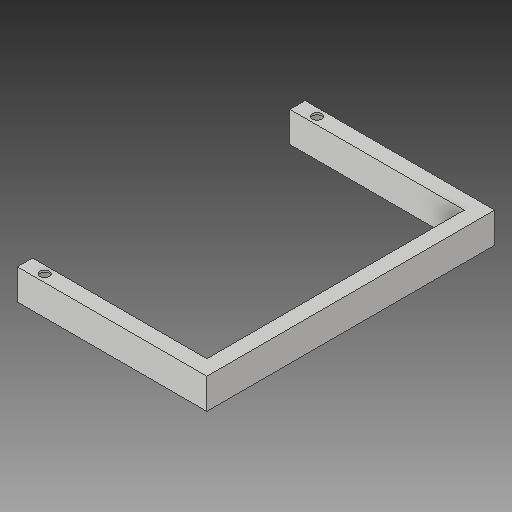
# Autodesk Inventor part: GripperFrame
Saved by Autodesk Inventor 2019 (Build 230136000, 136)
## iProperties
Created: 2018-01-17
Part Number: GripperFrame
Material: Generic
Document SubType Name: Modeling
Designer: steele
Density: 1 g/cm^3
Appearance: Default
Author: steele
Autodesk Inventor part; units mm, degrees
ref_plane "XZ Plane" through (0, 0, 0) normal (0, 1, 0) x (-1, 0, 0)
ref_plane "XY Plane" through (0, 0, 0) normal (0, 0, 1) x (1, 0, 0)
sketch "Sketch1" plane through (0, 0, 0) normal (0, 1, 0) x (-1, 0, 0)
  line L0 (304.8, -228.6) -> (0, -228.6)
  line L1 (0, -228.6) -> (0, 0)
  line L2 (0, 0) -> (304.8, 0) construction
  line L3 (304.8, 228.6) -> (0, 228.6)
  line L4 (0, 228.6) -> (0, 0)
  dimension "d0" = 304.8
  dimension "d1" = 228.6
  constraints: 10 end point, 2 horizontal, 2 symmetric about line, 1 perpendicular
  measures "d0" distance of L0.start L0.end
  measures "d1" distance of L0.end L1.end
ref_plane "Work Plane1" through (-304.8, 0, 0) normal (1, 0, 0) x (0, 1, 0)
sketch "Sketch2" plane through (-304.8, 0, 0) normal (1, 0, 0) x (0, 1, 0)
  line L0 (-25.4, -240.3674) -> (-25.4, -214.9674)
  line L1 (-25.4, -214.9674) -> (25.4, -214.9674)
  line L2 (25.4, -214.9674) -> (25.4, -240.3674)
  line L3 (25.4, -240.3674) -> (-25.4, -240.3674)
  line L4 (-25.4, -240.3674) -> (25.4, -214.9674) construction
  line L5 (-25.4, -214.9674) -> (25.4, -240.3674) construction
  line L6 (-22.225, -237.1924) -> (-22.225, -218.1424)
  line L7 (-22.225, -218.1424) -> (22.225, -218.1424)
  line L8 (22.225, -218.1424) -> (22.225, -237.1924)
  line L9 (22.225, -237.1924) -> (-22.225, -237.1924)
  line L10 (-22.225, -237.1924) -> (22.225, -218.1424) construction
  line L11 (-22.225, -218.1424) -> (22.225, -237.1924) construction
  point P0 (0, 0)
  point P1 (0, -227.6674)
  dimension "d3" = 25.4
  dimension "d4" = 50.8
  dimension "d5" = 3.175
  dimension "d6" = 3.175
  constraints: 24 end point, 4 midpoint, 4 parallel, 3 perpendicular, 1 vertical
  measures "d3" distance of L0.start L0.end
  measures "d4" distance of L0.end L1.end
  measures "d5" distance between parallel lines of L9 L3
  measures "d6" distance between parallel lines of L2 L8
sweep "Sweep1" add profiles "Sketch2" path "Sketch1"
sketch "Sketch3" plane through (-304.8, 25.4, -214.9674) normal (0, 1, 0) x (1, 0, 0)
  circle A0 centre (32.893, -442.6349) radius 7.9375
  line L0 (0, -455.3349) -> (0, -429.9349) projected
  point P0 (304.8, -214.9674)
  dimension "d9" = 15.875
  dimension "d10" = 32.893
  constraints: 1 centre point
  measures "d9" diameter of A0
  measures "d10" distance from line of A0.centre L0
extrude "Extrusion1" cut sketch "Sketch3" against normal through all
mirror "Mirror1" about plane through (0, 0, 0) normal (0, 0, 1) of "Extrusion1"
body "Solid1"
